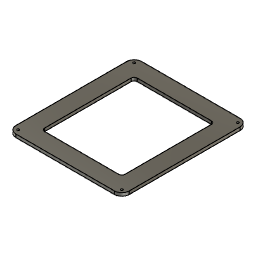
Top Cover Plate (Autodesk Fusion 360 design; units mm, degrees)
Autodesk Fusion 360 part; units mm, degrees
sketch "Sketch1" plane through (0, 0, 0) normal (0, 0, 1) x (1, 0, 0) in component "Top Cover Plate"
  line L0 (0, 0) -> (183.6, 0)
  line L1 (183.6, 0) -> (183.6, 203.6)
  line L2 (183.6, 203.6) -> (0, 203.6)
  line L3 (0, 203.6) -> (0, 0)
  dimension "d1" = 183.6
  dimension "d2" = 203.6
  constraint horizontal L0
  constraint vertical L1
  constraint horizontal L2
  constraint vertical L3
  constraint coincident L0.start L3.end
  measures "d1" distance of L0.start L0.end
  measures "d2" distance of L0.start L2.end
extrude "Extrude1" add sketch "Sketch1" along normal blind 5 in component "Top Cover Plate"
fillet "Fillet1" radius 12 4 edges at (183.6, 0, 2.5) (0, 0, 2.5) (183.6, 203.6, 2.5) (0, 203.6, 2.5) in component "Top Cover Plate"
sketch "Sketch2" plane through (0, 0, 5) normal (0, 0, 1) x (-1, 0, 0) in component "Top Cover Plate"
  arc A0 (-12, -203.6) -> (0, -191.6) centre (-12, -191.6) ccw
  line L0 (0, -191.6) -> (0, -12)
  arc A1 (0, -12) -> (-12, 0) centre (-12, -12) ccw
  line L1 (-12, 0) -> (-171.6, 0)
  arc A2 (-171.6, 0) -> (-183.6, -12) centre (-171.6, -12) ccw
  line L2 (-183.6, -12) -> (-183.6, -191.6)
  arc A3 (-183.6, -191.6) -> (-171.6, -203.6) centre (-171.6, -191.6) ccw
  line L3 (-171.6, -203.6) -> (-12, -203.6)
  line L4 (0, -195.8) -> (-183.6, -195.8) construction
  line L5 (0, -7.8) -> (-183.6, -7.8) construction
  line L6 (-7.8, -203.6) -> (-7.8, 0) construction
  line L7 (-175.8, -203.6) -> (-175.8, 0) construction
  circle A4 centre (-7.8, -195.8) radius 1.75
  circle A5 centre (-175.8, -195.8) radius 1.75
  circle A6 centre (-7.8, -7.8) radius 1.75
  circle A7 centre (-175.8, -7.8) radius 1.75
  dimension "d7" = 7.8
  dimension "d8" = 7.8
  dimension "d9" = 7.8
  dimension "d10" = 7.8
  dimension "d11" = 3.5
  dimension "d12" = 3.5
  dimension "d13" = 3.5
  dimension "d14" = 3.5
  constraint coincident L0 L4.start
  constraint coincident L2 L4.end
  constraint perpendicular L2 L4
  constraint coincident L0 L5.start
  constraint coincident L2 L5.end
  constraint perpendicular L2 L5
  constraint coincident L3 L6.start
  constraint coincident L1 L6.end
  constraint perpendicular L1 L6
  constraint coincident L3 L7.start
  constraint coincident L1 L7.end
  constraint perpendicular L1 L7
  constraint coincident L4 A4.centre
  constraint coincident L6 A4.centre
  constraint coincident L4 A5.centre
  constraint coincident L7 A5.centre
  constraint coincident L6 A6.centre
  constraint coincident L5 A6.centre
  constraint coincident L7 A7.centre
  constraint coincident L5 A7.centre
  measures "d7" distance of L3 L4
  measures "d8" distance of L0 L6
  measures "d9" distance of L1 L5
  measures "d10" distance of L2 L7
  measures "d11" diameter of A4
  measures "d12" diameter of A5
  measures "d13" diameter of A6
  measures "d14" diameter of A7
extrude "Extrude2" cut sketch "Sketch2" against normal up to surface (5 mm away) contours A4 | A5 | A6 | A7 in component "Top Cover Plate"
sketch "Sketch3" plane through (0, 0, 5) normal (0, 0, 1) x (-1, 0, 0) in component "Top Cover Plate"
  circle A0 centre (-175.8, -195.8) radius 1.75
  circle A1 centre (-7.8, -7.8) radius 1.75
  circle A2 centre (-7.8, -195.8) radius 1.75
  circle A3 centre (-175.8, -7.8) radius 1.75
  arc A4 (-12, -203.6) -> (0, -191.6) centre (-12, -191.6) ccw
  line L0 (0, -191.6) -> (0, -12)
  arc A5 (0, -12) -> (-12, 0) centre (-12, -12) ccw
  line L1 (-12, 0) -> (-171.6, 0)
  arc A6 (-171.6, 0) -> (-183.6, -12) centre (-171.6, -12) ccw
  line L2 (-183.6, -12) -> (-183.6, -191.6)
  arc A7 (-183.6, -191.6) -> (-171.6, -203.6) centre (-171.6, -191.6) ccw
  line L3 (-171.6, -203.6) -> (-12, -203.6)
  line L4 (-91.8, -203.6) -> (-91.8, 0) construction
  line L5 (0, -101.8) -> (-183.6, -101.8) construction
  line L6 (-156.8, -176.8) -> (-26.8, -176.8)
  line L7 (-26.8, -176.8) -> (-26.8, -26.8)
  line L8 (-26.8, -26.8) -> (-156.8, -26.8)
  line L9 (-156.8, -26.8) -> (-156.8, -176.8)
  line L10 (-156.8, -176.8) -> (-26.8, -26.8) construction
  line L11 (-26.8, -176.8) -> (-156.8, -26.8) construction
  point P0 (-91.8, -101.8)
  dimension "d17" = 130
  dimension "d18" = 150
  constraint midpoint L3 L4.start
  constraint midpoint L1 L4.end
  constraint midpoint L0 L5.start
  constraint midpoint L2 L5.end
  constraint horizontal L6
  constraint perpendicular L6 L7
  constraint parallel L6 L8
  constraint parallel L7 L9
  constraint coincident L10 P0
  constraint coincident L11 P0
  constraint midpoint L5 P0
  measures "d17" distance of L7.end L8.end
  measures "d18" distance of L6.end L7.end
extrude "Extrude3" cut sketch "Sketch3" against normal up to surface (5 mm away) contours L6 L7 L8 L9 in component "Top Cover Plate"
fillet "Fillet2" radius 5 4 edges at (26.8, 26.8, 2.5) (26.8, 176.8, 2.5) (156.8, 176.8, 2.5) (156.8, 26.8, 2.5) in component "Top Cover Plate"
component "Top Cover Plate" placed x (1, 0, 0) y (0, 1, 0) z (0, 0, 1) at (0, 0, 0)
